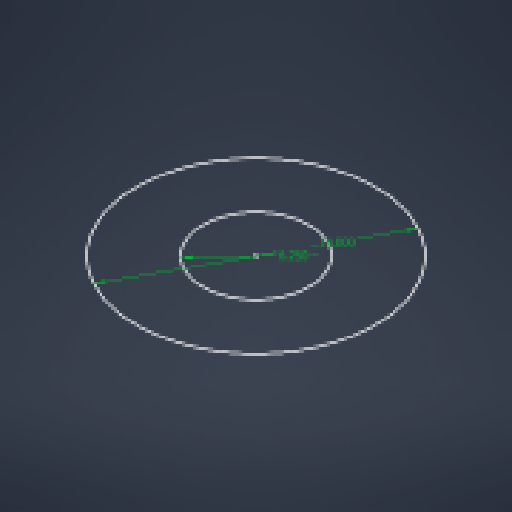
# Autodesk Inventor part: 3DPRINT,WIRE-GUARD
Saved by Autodesk Inventor 2026.1 (Build 301233020, 233B)
## iProperties
Created: 2026-03-02
Part Number: 3DPRINT,WIRE-GUARD
Material: Generic
Document SubType Name: Modeling
Designer: Owen L
Density: 1 g/cm^3
Appearance: Default
Mass: 47.0872 g
Surface Area: 1580.76 cm^2
Volume: 47.0872 cm^3
Author: Owen L
Autodesk Inventor part; units mm, degrees
ref_plane "YZ Plane" through (0, 0, 0) normal (1, 0, 0) x (0, 1, 0)
ref_plane "XZ Plane" through (0, 0, 0) normal (0, 1, 0) x (-1, 0, 0)
ref_plane "XY Plane" through (0, 0, 0) normal (0, 0, 1) x (1, 0, 0)
sketch "Sketch1" plane through (0, 0, 0) normal (0, 1, 0) x (-1, 0, 0)
  circle A0 centre (0, 0) radius 79.375
  circle A1 centre (0, 0) radius 177.8
  dimension "d0" = 158.75
  dimension "d1" = 355.6
  constraints: 2 centre point, 2 coincident
  measures "d0" diameter of A0
  measures "d1" diameter of A1
extrude "Extrusion1" add sketch "Sketch1" along normal blind 0.6
sketch "Sketch2" plane through (0, 0.6, 0) normal (0, 1, 0) x (1, 0, 0)
  point P0 (0, 0)
  point P1 (0, 90.4875)
  point P2 (-70.746, 56.418)
  point P3 (-88.2188, -20.1354)
  point P4 (-39.2611, -81.5264)
  point P5 (39.2611, -81.5264)
  point P6 (88.2188, -20.1354)
  point P7 (70.746, 56.418)
  dimension "d4" = 90.4875
  dimension "d7" = 360
  constraints: 1 vertical alignment, 8 other
  measures "d4" distance of point (0, 0) point (0, 90.487)
hole "Hole1" at (0, 0.6, -90.4875) at (-70.746, 0.6, -56.418) at (-88.2188, 0.6, 20.1354) at (-39.2611, 0.6, 81.5264) at (39.2611, 0.6, 81.5264) at (88.2188, 0.6, 20.1354) at (70.746, 0.6, -56.418) direction (0, -1, 0) diameter 6.7564 end through all clearance for "Hex Machine Screw" size "1/4" standard "Ansi Unified Screw Threads"
sketch "Sketch3" plane through (0, 0.6, 0) normal (0, 1, 0) x (1, 0, 0)
  point P0 (0, 0)
  point P1 (-143.51, 0)
  dimension "d16" = 143.51
  constraints: 1 horizontal alignment
  measures "d16" distance of point (0, 0) point (-143.51, 0)
hole "Hole2" at (-143.51, 0.6, 0) direction (0, -1, 0) diameter 31.75 end through all
body "Solid1"
